wheel mockup_v3 (Autodesk Fusion 360 design; units mm, degrees)
Autodesk Fusion 360 part; units mm, degrees
sketch "Sketch1" plane through (0, 0, 0) normal (0, 1, 0) x (1, 0, 0) in component "hub"
  circle A0 centre (0, 0) radius 25.75
  circle A1 centre (0, 0) radius 2.25
  circle A2 centre (0, 0) radius 22.25
  circle A3 centre (0, 0) radius 8
  line L0 (0, 0) -> (1.75, 0) construction
  line L1 (0, 0) -> (-1.75, 0) construction
  line L2 (-1.75, 0) -> (-1.75, -7.8062) construction
  line L3 (1.75, 0) -> (1.75, -7.8062) construction
  line L4 (-1.75, -7.8062) -> (-1.75, -22.1811)
  line L5 (1.75, -7.8062) -> (1.75, -22.1811)
  line L6 (2.3876, -7.6354) -> (9.575, -20.0844)
  line L7 (5.4187, -5.8854) -> (12.6061, -18.3344)
  line L8 (5.8854, -5.4187) -> (18.3344, -12.6061)
  line L9 (7.6354, -2.3876) -> (20.0844, -9.575)
  line L10 (7.8062, -1.75) -> (22.1811, -1.75)
  line L11 (7.8062, 1.75) -> (22.1811, 1.75)
  line L12 (7.6354, 2.3876) -> (20.0844, 9.575)
  line L13 (5.8854, 5.4187) -> (18.3344, 12.6061)
  line L14 (5.4187, 5.8854) -> (12.6061, 18.3344)
  line L15 (2.3876, 7.6354) -> (9.575, 20.0844)
  line L16 (1.75, 7.8062) -> (1.75, 22.1811)
  line L17 (-1.75, 7.8062) -> (-1.75, 22.1811)
  line L18 (-2.3876, 7.6354) -> (-9.575, 20.0844)
  line L19 (-5.4187, 5.8854) -> (-12.6061, 18.3344)
  line L20 (-5.8854, 5.4187) -> (-18.3344, 12.6061)
  line L21 (-7.6354, 2.3876) -> (-20.0844, 9.575)
  line L22 (-7.8062, 1.75) -> (-22.1811, 1.75)
  line L23 (-7.8062, -1.75) -> (-22.1811, -1.75)
  line L24 (-7.6354, -2.3876) -> (-20.0844, -9.575)
  line L25 (-5.8854, -5.4187) -> (-18.3344, -12.6061)
  line L26 (-5.4187, -5.8854) -> (-12.6061, -18.3344)
  line L27 (-2.3876, -7.6354) -> (-9.575, -20.0844)
  dimension "d28" = 51.5
  dimension "d29" = 4.5
  dimension "d30" = 44.5
  dimension "d33" = 16
  dimension "d40" = 1.75
  dimension "d41" = 1.75
  dimension "d43" = 360
  constraint coincident A0.centre A1.centre
  constraint concentric A1 A2
  constraint concentric A0 A3
  constraint horizontal L0
  constraint parallel L0 L1
  constraint coincident A3 L2.end
  constraint perpendicular L1 L2
  constraint coincident A3 L3.end
  constraint perpendicular L0 L3
  constraint coincident A2 L4.end
  constraint parallel L2 L4
  constraint coincident A2 L5.end
  constraint parallel L3 L5
  measures "d28" diameter of A0
  measures "d29" diameter of A1
  measures "d30" diameter of A2
  measures "d33" diameter of A3
  measures "d40" distance of A0.centre L0.end
  measures "d41" distance of A0.centre L1.end
extrude "Extrude1" add sketch "Sketch1" along normal blind 25.3 contours A0 makes body 1 in component "hub"
extrude "Extrude2" add sketch "Sketch1" along normal blind 6 from surface at 11 separate body contours A3 makes body 2 in component "hub"
sketch "Sketch2" plane through (0, 17, 0) normal (0, 1, 0) x (-1, 0, 0) in component "hub"
  circle A0 centre (0, 0) radius 2.25
  circle A1 centre (0, 0) radius 8
  line L0 (0, -7) -> (6.0622, -3.5)
  line L1 (6.0622, -3.5) -> (6.0622, 3.5)
  line L2 (6.0622, 3.5) -> (0, 7)
  line L3 (0, 7) -> (-6.0622, 3.5)
  line L4 (-6.0622, 3.5) -> (-6.0622, -3.5)
  line L5 (-6.0622, -3.5) -> (0, -7)
  dimension "d37" = 7
  constraint coincident A0.centre A1.centre
  constraint vertical L1
  measures "d37" distance of L0.start A0.centre
extrude "Extrude3" cut sketch "Sketch2" against normal blind 4.2 contours L0 L1 L2 L3 L4 L5 bodies 2 in component "hub"
extrude "Extrude4" add sketch "Sketch1" along normal up to surface (12.8 mm away) separate body contours A2 A3 L10 L11 | A2 A3 L12 L13 | A2 A3 L8 L9 | A2 A3 L14 L15 | A2 A3 L6 L7 | A2 A3 L16 L17 | A2 A3 L4 L5 | A2 A3 L18 L19 | A2 A3 L26 L27 | A2 A3 L20 L21 | A2 A3 L24 L25 | A2 A3 L22 L23 makes body 3 at (-7.8145, 4.2667, 10.0351) makes body 4 at (4.7834, 4.2667, 11.7851) makes body 5 at (4.7834, 4.2667, -11.7851) makes body 6 at (11.7851, 4.2667, -4.7834) makes body 7 at (10.0351, 4.2667, 7.8145) makes body 8 at (-11.7851, 8.5333, 4.7834) makes body 9 at (-12.5979, 8.5333, -1.75) makes body 10 at (12.5979, 8.5333, 1.75) makes body 11 at (-4.7834, 4.2667, -11.7851) makes body 12 at (1.75, 8.5333, -12.5979) makes body 13 at (-10.0351, 8.5333, -7.8145) makes body 14 at (-1.75, 8.5333, 12.5979) in component "hub"
chamfer "Chamfer1" distance 11 angle 45 12 edges at (6.9282, 0, -4) (6.9282, 0, 4) (-8, 0, 0) (-6.9282, 0, 4) (8, 0, 0) (0, 0, -8) (4, 0, -6.9282) (-4, 0, -6.9282) (0, 0, 8) (4, 0, 6.9282) (-4, 0, 6.9282) (-6.9282, 0, -4) on bodies 3 4 5 6 7 8 9 10 11 12 13 14 in component "hub"
chamfer "Chamfer1" distance 10 angle 45 11 edges at (19.2691, 12.8, -11.125) (19.2691, 12.8, 11.125) (-22.25, 12.8, 0) (-19.2691, 12.8, 11.125) (0, 12.8, -22.25) (11.125, 12.8, -19.2691) (-11.125, 12.8, -19.2691) (0, 12.8, 22.25) (11.125, 12.8, 19.2691) (-11.125, 12.8, 19.2691) (-19.2691, 12.8, -11.125) on bodies 3 4 5 6 7 8 9 10 11 12 13 14 in component "hub"
chamfer "Chamfer1" distance 10 angle 45 1 edges at (22.25, 12.8, 0) on bodies 3 4 5 6 7 8 9 10 11 12 13 14 in component "hub"
combine "Combine1" operation add target body 1 tool bodies 11 13 9 8 3 14 4 7 10 6 5 12 2 in component "hub"
sketch "Sketch1 (2)" plane through (0, 0, 0) normal (0, 1, 0) x (1, 0, 0) in component "Wheel"
  circle A0 centre (0, 0) radius 25.75
  circle A1 centre (0, 0) radius 33.75
  dimension "d49" = 67.5
  constraint concentric A0 A1
  measures "d49" diameter of A1
extrude "Extrude1'" add sketch "Sketch1 (2)" along normal up to surface (25.3 mm away) separate body makes body 15 in component "Wheel"
extrude "Extrude2'" add 1 faces at (30.8618, 25.3, 2.956) along direction (0, 1, 0) blind 1.25 on bodies 15 bodies 15 in component "Wheel"
extrude "Extrude3'" add 1 faces at (30.8618, 0, 2.956) along direction (0, -1, 0) blind 1.25 on bodies 15 bodies 15 in component "Wheel"
component "hub" placed x (1, 0, 0) y (0, 1, 0) z (0, 0, 1) at (0, 0, 0)
component "Wheel" placed x (1, 0, 0) y (0, 1, 0) z (0, 0, 1) at (0, 0, 0)
equation "d37 = ( 14 / 2 ) * 1 mm"
equation "d40 = ( 3.5 / 2 ) * 1 mm"
equation "d41 = d40"
equation "d52 = ( ( 27.5 - 25 ) / 2 ) * 1 mm"
equation "d54 = ( ( 27.5 - 25 ) / 2 ) * 1 mm"
